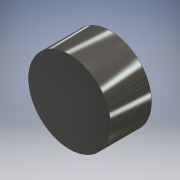
# Autodesk Inventor part: neodym_magnet
Saved by Autodesk Inventor 2016 (Build 200138000, 138)
## iProperties
Created: 2018-04-10
Part Number: neodym_magnet
Material: Nickel-Copper Alloy 400
Document SubType Name: Modeling
Designer: Eivind
Mass: 0.221922 g
Surface Area: 0.502655 cm^2
Volume: 0.0251327 cm^3
Density: 8.83 g/cm^3
Appearance: Chrome - Polished
Author: Eivind
Autodesk Inventor part; units mm, degrees
ref_plane "YZ Plane" through (0, 0, 0) normal (1, 0, 0) x (0, 1, 0)
ref_plane "XZ Plane" through (0, 0, 0) normal (0, 1, 0) x (-1, 0, 0)
ref_plane "XY Plane" through (0, 0, 0) normal (0, 0, 1) x (1, 0, 0)
sketch "Sketch1" plane through (0, 0, 0) normal (0, 1, 0) x (-1, 0, 0)
  circle A0 centre (0, 0) radius 2
  dimension "d0" = 4
  constraints: 1 centre point, 1 coincident
  measures "d0" diameter of A0
extrude "Extrusion1" add sketch "Sketch1" along normal blind 2
body "Solid1"
